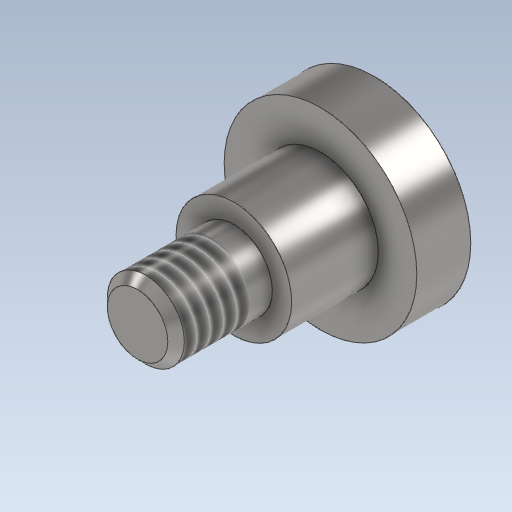
# Autodesk Inventor part: DBTS4-4.5-5-LTC
Saved by Autodesk Inventor 2020.4 (Build 244396000, 396)
## iProperties
Part Number: DBTS4-4.5-5-LTC
Material: ステンレス鋼 AISI 304
Document SubType Name: Modeling
Designer: Masato Kubotera
Density: 8 g/cm^3
Appearance: 半つや出し
Catalog Web Link: https://jp.misumi-ec.com/vona2/detail/110302679110/?HissuCode=DBTS4-4.5-5-LTC
Description: ReadyMade
Mass: 3.20624 g
Surface Area: 4.02284 cm^2
Volume: 0.40078 cm^3
Author: Masato Kubotera
Comments: Width across flats : 2
Autodesk Inventor part; units mm, degrees
ref_plane "YZ Plane" through (0, 0, 0) normal (1, 0, 0) x (0, 1, 0)
ref_plane "XZ Plane" through (0, 0, 0) normal (0, 1, 0) x (-1, 0, 0)
ref_plane "XY Plane" through (0, 0, 0) normal (0, 0, 1) x (1, 0, 0)
sketch "スケッチ1" plane through (0, 0, 0) normal (0, 1, 0) x (-1, 0, 0)
  line L0 (0, 0) -> (-5, 0)
  line L1 (-5, 0) -> (-5, 2.8)
  line L2 (-5, 2.8) -> (-3, 2.8)
  line L3 (-3, 2.8) -> (-3, 7.3)
  line L4 (-3, 7.3) -> (-2, 7.3)
  line L5 (-2, 7.3) -> (-2, 11.87)
  line L6 (-1.57, 12.3) -> (0, 12.3)
  line L7 (0, 12.3) -> (0, 0)
  line L8 (-1.57, 12.3) -> (-2, 11.87)
  point P0 (-2, 12.3)
  dimension "d0" = 5
  dimension "d1" = 4.5
  dimension "d2" = 2.8
  dimension "d3" = 0.43
  dimension "d4" = 0.43
  dimension "d5" = 4
  dimension "d6" = 10
  dimension "d7" = 6
  constraints: 18 end point, 7 perpendicular, 2 point on line, 1 horizontal
  measures "d0" distance of L4.end point (-2, 12.3)
  measures "d1" distance of L2.end L3.end
  measures "d2" distance of L0.end L1.end
  measures "d3" distance of L6.start point (-2, 12.3)
  measures "d4" distance of L5.end point (-2, 12.3)
  measures "d5" diameter of L5.end L7
  measures "d6" diameter of L0.end L7
  measures "d7" diameter of L2.end L7
revolve "回転1" add sketch "スケッチ1" angle 360 about axis through (0, 0, 12.3) along (0, 0, -1)
thread "ねじ1" size "M4x0.7" class "6g" standard "ANSI Metric M Profile" length 7.57 offset 1.2
sketch "スケッチ2" plane through (0, 0, 0) normal (0, 0, -1) x (-1, 0, 0)
  line L0 (0, -1.4434) -> (-1.25, -0.7217)
  line L1 (-1.25, -0.7217) -> (-1.25, 0.7217)
  line L2 (-1.25, 0.7217) -> (0, 1.4434)
  line L3 (0, 1.4434) -> (1.25, 0.7217)
  line L4 (1.25, 0.7217) -> (1.25, -0.7217)
  line L5 (1.25, -0.7217) -> (0, -1.4434)
  point P0 (0, 0)
  point P1 (0, 0)
  dimension "d11" = 2.5
  constraints: 12 end point, 1 coincident, 1 vertical, 13 other
  measures "d11" distance of L1.end L3.end
extrude "押し出し1" cut sketch "スケッチ2" against normal blind 1.5
equation "\"d4\" = d3"
